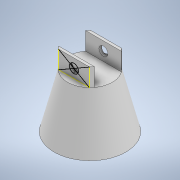
# Autodesk Inventor part: base
Saved by Autodesk Inventor 2020 (Build 240168000, 168)
## iProperties
Created: 2020-12-23
Part Number: base
Material: Generic
Document SubType Name: Modeling
Designer: frost
Density: 1 g/cm^3
Appearance: Default
Author: frost
Autodesk Inventor part; units mm, degrees
ref_plane "YZ Plane" through (0, 0, 0) normal (1, 0, 0) x (0, 1, 0)
ref_plane "XZ Plane" through (0, 0, 0) normal (0, 1, 0) x (-1, 0, 0)
ref_plane "XY Plane" through (0, 0, 0) normal (0, 0, 1) x (1, 0, 0)
sketch "Sketch1" plane through (0, 0, 0) normal (0, 0, 1) x (1, 0, 0)
  line L0 (0, 0) -> (0, -60)
  line L1 (0, -60) -> (-40, -60)
  line L2 (0, 0) -> (-25, 0)
  line L3 (-25, 0) -> (-40, -60)
  dimension "d0" = 40
  dimension "d1" = 25
  dimension "d2" = 60
  constraints: 8 end point, 1 horizontal, 1 perpendicular, 1 vertical
  measures "d0" distance of L0.end L1.end
  measures "d1" distance of L0.start L2.end
  measures "d2" distance of L0.start L0.end
revolve "Revolution1" add sketch "Sketch1" angle 360 about axis through (0, 0, 0) along (0, -1, 0)
sketch "Sketch2" plane through (0, 0, 0) normal (0, 1, 0) x (1, 0, 0)
  line L0 (0, 0) -> (0, 15)
  line L1 (0, 15) -> (-20, 15)
  circle A0 centre (0, 0) radius 25 projected
  line L2 (0, 15) -> (20, 15)
  line L3 (0, 0) -> (-17.5771, 0)
  line L4 (0, -15) -> (-20, -15)
  line L5 (0, -15) -> (20, -15)
  line L6 (-17.3494, -18) -> (17.3494, -18)
  line L7 (-17.3494, -18) -> (-20, -15)
  line L8 (20, -15) -> (17.3494, -18)
  line L9 (0, 0) -> (12.1648, 0)
  line L10 (-17.3494, 18) -> (17.3494, 18)
  line L11 (-17.3494, 18) -> (-20, 15)
  line L12 (20, 15) -> (17.3494, 18)
  dimension "d4" = 15
  dimension "d10" = 3
  constraints: 26 end point, 6 symmetric about line, 5 point on circle, 3 point on line, 2 horizontal, 1 perpendicular, 1 vertical
  measures "d4" distance of L0.start L0.end
  measures "d10" distance between parallel lines of L6 L5
extrude "Extrusion1" add sketch "Sketch2" along normal blind 20 contours L1 L11 L10 L12 L2 | L4 L5 L8 L6 L7
sketch "Sketch3" plane through (-17.3494, 0, 18) normal (0, 0, 1) x (1, 0, 0)
  line L0 (34.6987, 0) -> (34.6987, 20) projected
  line L1 (0, 0) -> (0, 20) projected
  line L2 (34.6987, 20) -> (0, 0)
  line L3 (34.6987, 0) -> (0, 0) projected
  line L4 (34.6987, 0) -> (0, 20)
  circle A0 centre (17.3494, 10) radius 5
  point P0 (17.3494, 0)
  dimension "d7" = 10
  constraints: 4 end point, 1 centre point, 1 midpoint
  measures "d7" diameter of A0
extrude "Extrusion2" cut sketch "Sketch3" against normal blind 60 contours A0 L2 L4 | L4 L2 A0 | L2 L4 A0 | A0 L4 L2
body "Solid1"
